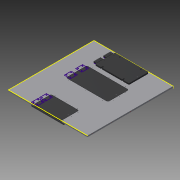
# Autodesk Inventor part: Front_part
Saved by Autodesk Inventor 2015 SP2 (Build 190223200, 223)
## iProperties
Created: 2016-11-11
Part Number: Front_part
Material: Generic
Document SubType Name: Modeling
Designer: Yann Cesbron
Density: 1 g/cm^3
Appearance: Default
Mass: 4194.72 g
Surface Area: 9649.71 cm^2
Volume: 4194.72 cm^3
Material: Perspex Black 9961 -10 mm
Author: Yann Cesbron
Autodesk Inventor part; units mm, degrees
(part 1 of 2)
ref_plane "YZ Plane" through (0, 0, 0) normal (1, 0, 0) x (0, 1, 0)
ref_plane "XZ Plane" through (0, 0, 0) normal (0, 1, 0) x (-1, 0, 0)
ref_plane "XY Plane" through (0, 0, 0) normal (0, 0, 1) x (1, 0, 0)
sketch "Sketch1" plane through (0, 0, 0) normal (0, 0, 1) x (1, 0, 0)
  line L0 (0, 0) -> (565, 0)
  line L1 (565, 0) -> (565, 610)
  line L2 (565, 610) -> (0, 610)
  line L3 (0, 610) -> (0, 0)
  dimension "d0" = 565
  dimension "d1" = 610
  constraints: 8 end point, 2 parallel, 1 horizontal, 1 perpendicular
  measures "d0" distance of L2.end L1.end
  measures "d1" distance of L1.end L0.end
extrude "Extrusion1" add sketch "Sketch1" along normal blind 10
sketch "Cut_out_front" plane through (0, 0, 10) normal (0, 0, 1) x (1, 0, 0)
  line L0 (180, 0) -> (380, 0)
  line L1 (380, 0) -> (380, 115)
  line L2 (370, 125) -> (190, 125)
  line L3 (180, 115) -> (180, 0)
  arc A0 (380, 115) -> (370, 125) centre (370, 115) ccw
  arc A1 (190, 125) -> (180, 115) centre (190, 115) ccw
  line L4 (140, 280) -> (420, 280)
  line L5 (430, 290) -> (430, 420)
  line L6 (420, 430) -> (140, 430)
  line L7 (130, 420) -> (130, 290)
  arc A2 (130, 290) -> (140, 280) centre (140, 290) ccw
  arc A3 (140, 430) -> (130, 420) centre (140, 420) ccw
  arc A4 (430, 420) -> (420, 430) centre (420, 420) ccw
  arc A5 (420, 280) -> (430, 290) centre (420, 290) ccw
  line L8 (0, 610) -> (0, 0) projected
  line L9 (0, 0) -> (565, 0) projected
  line L10 (565, 610) -> (0, 610) projected
  circle A6 centre (117.3, 411.4) radius 1.65
  circle A7 centre (117.3, 379.6) radius 1.65
  circle A8 centre (117.3, 330.4) radius 1.65
  circle A9 centre (117.3, 298.6) radius 1.65
  circle A10 centre (167.3, 13.6) radius 1.65
  circle A11 centre (167.3, 45.4) radius 1.65
  circle A12 centre (167.3, 72.1) radius 1.65
  circle A13 centre (167.3, 103.9) radius 1.65
  line L11 (185, 580) -> (375, 580)
  line L12 (380, 575) -> (380, 485)
  line L13 (375, 480) -> (185, 480)
  line L14 (180, 485) -> (180, 575)
  circle A14 centre (205, 590) radius 2.5
  circle A15 centre (355, 590) radius 2.5
  circle A16 centre (355, 470) radius 2.5
  circle A17 centre (205, 470) radius 2.5
  circle A18 centre (172.5, 565) radius 1.65
  circle A19 centre (172.5, 495) radius 1.65
  circle A20 centre (387.5, 565) radius 1.65
  circle A21 centre (387.5, 495) radius 1.65
  circle A22 centre (122.5, 355) radius 1.65
  circle A23 centre (122.5, 310) radius 1.65
  circle A24 centre (122.5, 400) radius 1.65
  circle A25 centre (160, 272.5) radius 1.65
  circle A26 centre (280, 272.5) radius 1.65
  circle A27 centre (400, 272.5) radius 1.65
  circle A28 centre (437.5, 310) radius 1.65
  circle A29 centre (437.5, 355) radius 1.65
  circle A30 centre (437.5, 400) radius 1.65
  circle A31 centre (400, 437.5) radius 1.65
  circle A32 centre (280, 437.5) radius 1.65
  circle A33 centre (160, 437.5) radius 1.65
  circle A34 centre (172.5, 7.5) radius 1.65
  circle A35 centre (172.5, 62.5) radius 1.65
  circle A36 centre (172.5, 110) radius 1.65
  circle A37 centre (280, 132.5) radius 1.65
  circle A38 centre (387.5, 110) radius 1.65
  circle A39 centre (387.5, 62.5) radius 1.65
  circle A40 centre (387.5, 7.5) radius 1.65
  arc A41 (380, 575) -> (375, 580) centre (375, 575) ccw
  arc A42 (375, 480) -> (380, 485) centre (375, 485) ccw
  arc A43 (180, 485) -> (185, 480) centre (185, 485) ccw
  arc A44 (185, 580) -> (180, 575) centre (185, 575) ccw
  circle A45 centre (200, 132.5) radius 1.65
  circle A46 centre (360, 132.5) radius 1.65
  point P0 (380, 125)
  point P1 (180, 125)
  point P2 (430, 430)
  point P3 (430, 280)
  point P4 (130, 430)
  point P5 (380, 480)
  point P6 (380, 580)
  point P7 (180, 480)
  dimension "d21" = 200
  dimension "d22" = 125
  dimension "d23" = 10
  dimension "d24" = 10
  dimension "d25" = 300
  dimension "d26" = 150
  dimension "d27" = 10
  dimension "d31" = 180
  dimension "d32" = 130
  dimension "d34" = 280
  dimension "d36" = 3.3
  dimension "d37" = 3.3
  dimension "d38" = 3.3
  dimension "d39" = 3.3
  dimension "d40" = 12.7
  dimension "d41" = 12.7
  dimension "d42" = 12.7
  dimension "d43" = 12.7
  dimension "d44" = 31.8
  dimension "d45" = 31.8
  dimension "d87" = 18.6
  dimension "d88" = 18.6
  dimension "d126" = 3.3
  dimension "d127" = 3.3
  dimension "d128" = 3.3
  dimension "d129" = 3.3
  dimension "d130" = 12.7
  dimension "d131" = 12.7
  dimension "d132" = 12.7
  dimension "d133" = 12.7
  dimension "d134" = 21.1
  dimension "d135" = 31.8
  dimension "d136" = 13.6
  dimension "d137" = 31.8
  dimension "d142" = 200
  dimension "d143" = 100
  dimension "d144" = 30
  dimension "d145" = 180
  dimension "d148" = 5
  dimension "d149" = 5
  dimension "d150" = 5
  dimension "d151" = 5
  dimension "d152" = 10
  dimension "d153" = 10
  dimension "d154" = 10
  dimension "d155" = 10
  dimension "d156" = 25
  dimension "d157" = 25
  dimension "d158" = 25
  dimension "d159" = 25
  dimension "d160" = 3.3
  dimension "d161" = 3.3
  dimension "d162" = 3.3
  dimension "d163" = 3.3
  dimension "d164" = 7.5
  dimension "d165" = 7.5
  dimension "d166" = 7.5
  dimension "d167" = 7.5
  dimension "d168" = 15
  dimension "d169" = 15
  dimension "d170" = 15
  dimension "d171" = 15
  dimension "d188" = 3.3
  dimension "d189" = 3.3
  constraints: 47 centre point, 24 end point, 20 point on circle, 20 tangent, 16 point on line, 7 parallel, 6 equal radius, 3 horizontal, 3 perpendicular, 1 collinear
  measures "d21" distance of point (180, 125) point (380, 125)
  measures "d22" distance of point (380, 125) L1.start
  measures "d23" radius of A0
  measures "d24" radius of A1
  measures "d25" distance of point (130, 430) point (430, 430)
  measures "d26" distance of point (430, 430) point (430, 280)
  measures "d27" radius of A2
  measures "d31" distance between parallel lines of L8 L3
  measures "d32" distance between parallel lines of L8 L7
  measures "d34" distance between parallel lines of L9 L4
  measures "d36" diameter of A6
  measures "d37" diameter of A7
  measures "d38" diameter of A8
  measures "d39" diameter of A9
  measures "d40" distance from line of L7 A6.centre
  measures "d41" distance from line of L7 A7.centre
  measures "d42" distance from line of L7 A8.centre
  measures "d43" distance from line of L7 A9.centre
  measures "d44" distance of A7.centre A6.centre
  measures "d45" distance of A9.centre A8.centre
  measures "d87" distance from line of L6 A6.centre
  measures "d88" distance from line of L4 A9.centre
  measures "d126" diameter of A10
  measures "d127" diameter of A11
  measures "d128" diameter of A12
  measures "d129" diameter of A13
  measures "d130" distance from line of L3 A13.centre
  measures "d131" distance from line of L3 A12.centre
  measures "d132" distance from line of L3 A11.centre
  measures "d133" distance from line of L3 A10.centre
  measures "d134" distance from line of L2 A13.centre
  measures "d135" distance of A12.centre A13.centre
  measures "d136" distance from line of L9 A10.centre
  measures "d137" distance of A11.centre A10.centre
  measures "d142" distance of point (380, 480) point (180, 480)
  measures "d143" distance of point (380, 580) point (380, 480)
  measures "d144" distance between parallel lines of L10 L11
  measures "d145" distance between parallel lines of L8 L14
  measures "d148" diameter of A14
  measures "d149" diameter of A15
  measures "d150" diameter of A16
  measures "d151" diameter of A17
  measures "d152" distance from line of L11 A14.centre
  measures "d153" distance from line of L11 A15.centre
  measures "d154" distance from line of L13 A17.centre
  measures "d155" distance from line of L13 A16.centre
  measures "d156" distance from line of A14.centre L14
  measures "d157" distance from line of L12 A15.centre
  measures "d158" distance from line of L12 A16.centre
  measures "d159" distance from line of L14 A17.centre
  measures "d160" diameter of A18
  measures "d161" diameter of A19
  measures "d162" diameter of A20
  measures "d163" diameter of A21
  measures "d164" distance from line of L14 A18.centre
  measures "d165" distance from line of L14 A19.centre
  measures "d166" distance from line of L12 A21.centre
  measures "d167" distance from line of L12 A20.centre
  measures "d168" distance from line of L11 A20.centre
  measures "d169" distance from line of L13 A21.centre
  measures "d170" distance from line of L13 A19.centre
  measures "d171" distance from line of L11 A18.centre
  measures "d188" diameter of A22
  measures "d189" diameter of A23
sketch "Windows_front" plane through (0, 0, 0) normal (0, 0, -1) x (-1, 0, 0)
  line L0 (-395, 585) -> (-165, 585)
  line L1 (-165, 585) -> (-165, 475)
  line L2 (-165, 475) -> (-395, 475)
  line L3 (-395, 585) -> (-165, 475) construction
  line L4 (-165, 585) -> (-395, 475) construction
  line L5 (0, 610) -> (0, 0) projected
  line L6 (-565, 610) -> (0, 610) projected
  line L7 (-395, 535) -> (-385, 535)
  line L8 (-385, 535) -> (-385, 525)
  line L9 (-385, 525) -> (-395, 525)
  line L10 (-395, 475) -> (-395, 525)
  line L11 (-395, 535) -> (-395, 585)
  point P0 (-280, 530)
  dimension "d184" = 230
  dimension "d185" = 110
  dimension "d186" = 280
  dimension "d187" = 80
  dimension "d821" = 10
  dimension "d822" = 50
  dimension "d824" = 10
  dimension "d825" = 10
  constraints: 20 end point, 4 parallel, 2 horizontal, 2 midpoint, 2 perpendicular
  measures "d184" distance of L1.end L2.end
  measures "d185" distance of L0.end L1.end
  measures "d186" distance from line of L5 point (-280, 530)
  measures "d187" distance from line of L6 point (-280, 530)
  measures "d821" distance of L7.end L8.end
  measures "d822" distance between parallel lines of L0 L7
  measures "d824" distance between parallel lines of L11 L8
  measures "d825" distance between parallel lines of L10 L8
sketch "Hinges_middle_bottom_front" plane through (0, 0, 10) normal (0, 0, 1) x (1, 0, 0)
  line L0 (108, 420) -> (152, 420)
  line L1 (152, 420) -> (152, 371)
  line L2 (152, 371) -> (108, 371)
  line L3 (108, 371) -> (108, 420)
  line L4 (108, 290) -> (152, 290)
  line L5 (152, 290) -> (152, 339)
  line L6 (152, 339) -> (108, 339)
  line L7 (108, 339) -> (108, 290)
  line L8 (0, 610) -> (0, 0) projected
  line L9 (0, 0) -> (565, 0) projected
  circle A0 centre (117.3, 411.4) radius 2.25
  circle A1 centre (117.3, 379.6) radius 2.25
  circle A2 centre (117.3, 330.4) radius 2.25
  circle A3 centre (117.3, 298.6) radius 2.25
  circle A4 centre (142.7, 411.4) radius 2.25
  circle A5 centre (142.7, 379.6) radius 2.25
  circle A6 centre (142.7, 330.4) radius 2.25
  circle A7 centre (142.7, 298.6) radius 2.25
  line L10 (158, 112.5) -> (202, 112.5)
  line L11 (202, 112.5) -> (202, 63.5)
  line L12 (202, 63.5) -> (158, 63.5)
  line L13 (158, 63.5) -> (158, 112.5)
  line L14 (158, 54) -> (202, 54)
  line L15 (202, 54) -> (202, 5)
  line L16 (202, 5) -> (158, 5)
  line L17 (158, 5) -> (158, 54)
  circle A8 centre (167.3, 103.9) radius 2.25
  circle A9 centre (167.3, 72.1) radius 2.25
  circle A10 centre (192.7, 103.9) radius 2.25
  circle A11 centre (192.7, 72.1) radius 2.25
  circle A12 centre (167.3, 45.4) radius 2.25
  circle A13 centre (192.7, 45.4) radius 2.25
  circle A14 centre (167.3, 13.6) radius 2.25
  circle A15 centre (192.7, 13.6) radius 2.25
  dimension "d56" = 44
  dimension "d57" = 49
  dimension "d58" = 44
  dimension "d59" = 49
  dimension "d60" = 108
  dimension "d61" = 290
  dimension "d62" = 371
  dimension "d63" = 4.5
  dimension "d64" = 4.5
  dimension "d65" = 4.5
  dimension "d66" = 4.5
  dimension "d67" = 4.5
  dimension "d68" = 4.5
  dimension "d69" = 4.5
  dimension "d70" = 4.5
  dimension "d71" = 9.3
  dimension "d72" = 9.3
  dimension "d73" = 9.3
  dimension "d74" = 9.3
  dimension "d75" = 9.3
  dimension "d76" = 8.6
  dimension "d77" = 8.6
  dimension "d78" = 8.6
  dimension "d79" = 8.6
  dimension "d80" = 8.6
  dimension "d81" = 8.6
  dimension "d82" = 8.6
  dimension "d83" = 8.6
  dimension "d84" = 9.3
  dimension "d85" = 9.3
  dimension "d86" = 9.3
  dimension "d89" = 44
  dimension "d90" = 49
  dimension "d91" = 44
  dimension "d92" = 49
  dimension "d93" = 5
  dimension "d96" = 112.5
  dimension "d100" = 158
  dimension "d101" = 158
  dimension "d102" = 4.5
  dimension "d103" = 4.5
  dimension "d104" = 4.5
  dimension "d105" = 4.5
  dimension "d106" = 4.5
  dimension "d107" = 4.5
  dimension "d108" = 4.5
  dimension "d109" = 4.5
  dimension "d110" = 8.6
  dimension "d111" = 8.6
  dimension "d112" = 8.6
  dimension "d113" = 8.6
  dimension "d114" = 8.6
  dimension "d115" = 8.6
  dimension "d116" = 8.6
  dimension "d117" = 8.6
  dimension "d118" = 9.3
  dimension "d119" = 9.3
  dimension "d120" = 9.3
  dimension "d121" = 9.3
  dimension "d122" = 9.3
  dimension "d123" = 9.3
  dimension "d124" = 9.3
  dimension "d125" = 9.3
  constraints: 32 end point, 16 centre point, 8 parallel, 4 horizontal, 4 perpendicular, 1 point on line
  measures "d56" distance of L1.end L2.end
  measures "d57" distance of L0.end L1.end
  measures "d58" distance of L6.end L5.end
  measures "d59" distance of L5.end L4.end
  measures "d60" distance between parallel lines of L8 L3
  measures "d61" distance between parallel lines of L9 L4
  measures "d62" distance between parallel lines of L9 L2
  measures "d63" diameter of A0
  measures "d64" diameter of A1
  measures "d65" diameter of A2
  measures "d66" diameter of A3
  measures "d67" diameter of A4
  measures "d68" diameter of A5
  measures "d69" diameter of A6
  measures "d70" diameter of A7
  measures "d71" distance from line of L1 A5.centre
  measures "d72" distance from line of L1 A4.centre
  measures "d73" distance from line of L5 A6.centre
  measures "d74" distance from line of L3 A0.centre
  measures "d75" distance from line of L3 A1.centre
  measures "d76" distance from line of L0 A0.centre
  measures "d77" distance from line of L2 A1.centre
  measures "d78" distance from line of L2 A5.centre
  measures "d79" distance from line of L0 A4.centre
  measures "d80" distance from line of L6 A2.centre
  measures "d81" distance from line of L6 A6.centre
  measures "d82" distance from line of L4 A3.centre
  measures "d83" distance from line of L4 A7.centre
  measures "d84" distance from line of L7 A2.centre
  measures "d85" distance from line of L7 A3.centre
  measures "d86" distance from line of L5 A7.centre
  measures "d89" distance of L11.end L12.end
  measures "d90" distance of L10.end L11.end
  measures "d91" distance of L15.end L16.end
  measures "d92" distance of L14.end L15.end
  measures "d93" distance between parallel lines of L9 L16
  measures "d96" distance between parallel lines of L9 L10
  measures "d100" distance between parallel lines of L8 L13
  measures "d101" distance between parallel lines of L8 L17
  measures "d102" diameter of A8
  measures "d103" diameter of A9
  measures "d104" diameter of A10
  measures "d105" diameter of A11
  measures "d106" diameter of A12
  measures "d107" diameter of A13
  measures "d108" diameter of A14
  measures "d109" diameter of A15
  measures "d110" distance from line of L10 A8.centre
  measures "d111" distance from line of L10 A10.centre
  measures "d112" distance from line of L12 A9.centre
  measures "d113" distance from line of L12 A11.centre
  measures "d114" distance from line of A12.centre L14
  measures "d115" distance from line of L14 A13.centre
  measures "d116" distance from line of L16 A14.centre
  measures "d117" distance from line of L16 A15.centre
  measures "d118" distance from line of L13 A9.centre
  measures "d119" distance from line of L13 A8.centre
  measures "d120" distance from line of L11 A10.centre
  measures "d121" distance from line of L11 A11.centre
  measures "d122" distance from line of L15 A13.centre
  measures "d123" distance from line of L15 A15.centre
  measures "d124" distance from line of L17 A14.centre
  measures "d125" distance from line of L17 A12.centre
sketch "Top_door_hinge_levellers_front" plane through (0, 0, 10) normal (0, 0, 1) x (1, 0, 0)
  line L0 (158, 540.5) -> (138, 540.5)
  line L1 (138, 540.5) -> (138, 589.5)
  line L2 (138, 589.5) -> (158, 589.5)
  line L3 (158, 589.5) -> (158, 540.5)
  line L4 (138, 519.5) -> (158, 519.5)
  line L5 (158, 519.5) -> (158, 470.5)
  line L6 (158, 470.5) -> (138, 470.5)
  line L7 (138, 470.5) -> (138, 519.5)
  line L8 (565, 610) -> (0, 610) projected
  line L9 (0, 610) -> (0, 0) projected
  circle A0 centre (147.3, 580.9) radius 1.65
  circle A1 centre (147.3, 549.1) radius 1.65
  circle A2 centre (147.3, 479.1) radius 1.65
  circle A3 centre (147.3, 510.9) radius 1.65
  dimension "d304" = 20
  dimension "d305" = 49
  dimension "d306" = 20
  dimension "d307" = 49
  dimension "d308" = 20.5
  dimension "d309" = 139.5
  dimension "d310" = 138
  dimension "d311" = 138
  dimension "d312" = 3.3
  dimension "d313" = 3.3
  dimension "d314" = 3.3
  dimension "d315" = 3.3
  dimension "d316" = 8.6
  dimension "d317" = 8.6
  dimension "d318" = 9.3
  dimension "d319" = 9.3
  dimension "d320" = 9.3
  dimension "d321" = 9.3
  dimension "d322" = 8.6
  dimension "d323" = 8.6
  constraints: 16 end point, 4 centre point, 4 parallel, 2 horizontal, 2 perpendicular
  measures "d304" distance of L1.end L2.end
  measures "d305" distance of L0.end L1.end
  measures "d306" distance of L5.end L6.end
  measures "d307" distance of L4.end L5.end
  measures "d308" distance between parallel lines of L8 L2
  measures "d309" distance between parallel lines of L6 L8
  measures "d310" distance between parallel lines of L9 L1
  measures "d311" distance between parallel lines of L9 L7
  measures "d312" diameter of A0
  measures "d313" diameter of A1
  measures "d314" diameter of A2
  measures "d315" diameter of A3
  measures "d316" distance from line of L2 A0.centre
  measures "d317" distance from line of L0 A1.centre
  measures "d318" distance from line of L1 A1.centre
  measures "d319" distance from line of A0.centre L1
  measures "d320" distance from line of L7 A2.centre
  measures "d321" distance from line of L7 A3.centre
  measures "d322" distance from line of L4 A3.centre
  measures "d323" distance from line of L6 A2.centre
sketch "Top_door_front" plane through (0, 0, 10) normal (0, 0, 1) x (1, 0, 0)
  line L0 (165, 600) -> (395, 600)
  line L1 (400, 595) -> (400, 465)
  line L2 (160, 465) -> (160, 595)
  line L3 (160, 600) -> (400, 460) construction
  line L4 (400, 600) -> (160, 460) construction
  line L5 (565, 610) -> (0, 610) projected
  line L6 (0, 610) -> (0, 0) projected
  arc A0 (208.5, 470) -> (201.5, 470) centre (205, 470) ccw
  arc A1 (358.5, 470) -> (351.5, 470) centre (355, 470) ccw
  circle A2 centre (355, 590) radius 4
  circle A3 centre (205, 590) radius 4
  line L7 (201.5, 470) -> (201.5, 460)
  line L8 (208.5, 470) -> (208.5, 460)
  line L9 (351.5, 470) -> (351.5, 460)
  line L10 (358.5, 470) -> (358.5, 460)
  line L11 (395, 460) -> (358.5, 460)
  line L12 (351.5, 460) -> (208.5, 460)
  line L13 (201.5, 460) -> (165, 460)
  circle A4 centre (172.7, 580.9) radius 1.65
  circle A5 centre (172.7, 549.1) radius 1.65
  circle A6 centre (172.7, 510.9) radius 1.65
  circle A7 centre (172.7, 479.1) radius 1.65
  arc A8 (400, 595) -> (395, 600) centre (395, 595) ccw
  arc A9 (165, 600) -> (160, 595) centre (165, 595) ccw
  arc A10 (160, 465) -> (165, 460) centre (165, 465) ccw
  arc A11 (395, 460) -> (400, 465) centre (395, 465) ccw
  point P0 (280, 530)
  dimension "d138" = 240
  dimension "d139" = 140
  dimension "d146" = 280
  dimension "d147" = 80
  dimension "d172" = 7
  dimension "d173" = 7
  dimension "d174" = 8
  dimension "d175" = 8
  dimension "d176" = 10
  dimension "d177" = 10
  dimension "d180" = 45
  dimension "d181" = 45
  dimension "d182" = 45
  dimension "d183" = 45
  dimension "d299" = 10
  dimension "d300" = 10
  dimension "d301" = 150
  dimension "d302" = 10
  dimension "d388" = 3.3
  dimension "d389" = 3.3
  dimension "d390" = 3.3
  dimension "d391" = 3.3
  dimension "d392" = 19.1
  dimension "d393" = 31.8
  dimension "d394" = 31.8
  dimension "d395" = 19.1
  dimension "d396" = 12.7
  dimension "d397" = 12.7
  dimension "d398" = 12.7
  dimension "d399" = 12.7
  dimension "d400" = 5
  dimension "d401" = 5
  dimension "d402" = 5
  constraints: 24 end point, 13 perpendicular, 12 centre point, 12 point on circle, 12 tangent, 8 point on line, 4 parallel, 2 midpoint, 1 equal radius, 1 horizontal
  measures "d138" distance of L3.end L4.end
  measures "d139" distance of L4.start L3.end
  measures "d146" distance from line of L6 point (280, 530)
  measures "d147" distance from line of L5 point (280, 530)
  measures "d172" diameter of A0
  measures "d173" diameter of A1
  measures "d174" diameter of A2
  measures "d175" diameter of A3
  measures "d176" distance from line of L0 A2.centre
  measures "d177" distance from line of L0 A3.centre
  measures "d180" distance from line of L2 A3.centre
  measures "d181" distance from line of L1 A2.centre
  measures "d182" distance from line of L1 A1.centre
  measures "d183" distance from line of L2 A0.centre
  measures "d299" distance from line of L12 A1.centre
  measures "d300" distance from line of L12 A0.centre
  measures "d301" distance between parallel lines of L5 L12
  measures "d302" distance between parallel lines of L5 L0
  measures "d388" diameter of A4
  measures "d389" diameter of A5
  measures "d390" diameter of A6
  measures "d391" diameter of A7
  measures "d392" distance from line of L13 A7.centre
  measures "d393" distance of A6.centre A7.centre
  measures "d394" distance of A4.centre A5.centre
  measures "d395" distance from line of L0 A4.centre
  measures "d396" distance from line of L2 A7.centre
  measures "d397" distance from line of L2 A6.centre
  measures "d398" distance from line of L2 A5.centre
  measures "d399" distance from line of L2 A4.centre
  measures "d400" radius of A8
  measures "d401" radius of A9
  measures "d402" radius of A10
sketch "Hinges_top_front" plane through (0, 0, 10) normal (0, 0, 1) x (1, 0, 0)
  line L0 (182, 519.5) -> (182, 470.5)
  circle A0 centre (172.7, 510.9) radius 2.25
  circle A1 centre (172.7, 479.1) radius 2.25
  circle A2 centre (147.3, 479.1) radius 2.25
  circle A3 centre (147.3, 510.9) radius 2.25
  line L1 (182, 470.5) -> (138, 470.5)
  line L2 (138, 470.5) -> (138, 519.5)
  line L3 (138, 519.5) -> (182, 519.5)
  line L4 (182, 589.5) -> (182, 540.5)
  circle A4 centre (172.7, 580.9) radius 2.25
  circle A5 centre (172.7, 549.1) radius 2.25
  circle A6 centre (147.3, 549.1) radius 2.25
  circle A7 centre (147.3, 580.9) radius 2.25
  line L5 (182, 540.5) -> (138, 540.5)
  line L6 (138, 540.5) -> (138, 589.5)
  line L7 (138, 589.5) -> (182, 589.5)
  line L8 (0, 610) -> (0, 0) projected
  line L9 (565, 610) -> (0, 610) projected
  dimension "d356" = 44
  dimension "d357" = 49
  dimension "d358" = 4.5
  dimension "d359" = 4.5
  dimension "d360" = 4.5
  dimension "d361" = 4.5
  dimension "d362" = 9.3
  dimension "d363" = 9.3
  dimension "d364" = 9.3
  dimension "d365" = 9.3
  dimension "d366" = 8.6
  dimension "d367" = 8.6
  dimension "d368" = 8.6
  dimension "d369" = 8.6
  dimension "d370" = 44
  dimension "d371" = 49
  dimension "d372" = 4.5
  dimension "d373" = 4.5
  dimension "d374" = 4.5
  dimension "d375" = 4.5
  dimension "d376" = 9.3
  dimension "d377" = 9.3
  dimension "d378" = 9.3
  dimension "d379" = 9.3
  dimension "d380" = 8.6
  dimension "d381" = 8.6
  dimension "d382" = 8.6
  dimension "d383" = 8.6
  dimension "d384" = 138
  dimension "d385" = 138
  dimension "d386" = 20.5
  dimension "d387" = 139.5
  constraints: 16 end point, 8 centre point, 4 parallel, 2 horizontal, 2 perpendicular
  measures "d356" distance of L2.end L0.start
  measures "d357" distance of L1.end L2.end
  measures "d358" diameter of A0
  measures "d359" diameter of A1
  measures "d360" diameter of A2
  measures "d361" diameter of A3
  measures "d362" distance from line of L0 A1.centre
  measures "d363" distance from line of L0 A0.centre
  measures "d364" distance from line of L2 A3.centre
  measures "d365" distance from line of A2.centre L2
  measures "d366" distance from line of L1 A2.centre
  measures "d367" distance from line of L1 A1.centre
  measures "d368" distance from line of L3 A0.centre
  measures "d369" distance from line of L3 A3.centre
  measures "d370" distance of L6.end L4.start
  measures "d371" distance of L5.end L6.end
  measures "d372" diameter of A4
  measures "d373" diameter of A5
  measures "d374" diameter of A6
  measures "d375" diameter of A7
  measures "d376" distance from line of L4 A5.centre
  measures "d377" distance from line of L4 A4.centre
  measures "d378" distance from line of L6 A7.centre
  measures "d379" distance from line of A6.centre L6
  measures "d380" distance from line of L5 A6.centre
  measures "d381" distance from line of L5 A5.centre
  measures "d382" distance from line of L7 A4.centre
  measures "d383" distance from line of L7 A7.centre
  measures "d384" distance between parallel lines of L8 L2
  measures "d385" distance between parallel lines of L8 L6
  measures "d386" distance between parallel lines of L9 L7
  measures "d387" distance between parallel lines of L9 L1
sketch "Middle_door_front" plane through (0, 0, 10) normal (0, 0, 1) x (1, 0, 0)
  line L0 (140, 282) -> (420, 282)
  line L1 (428, 290) -> (428, 420)
  line L2 (420, 428) -> (140, 428)
  line L3 (132, 420) -> (132, 290)
  line L4 (132, 282) -> (428, 428) construction
  line L5 (428, 282) -> (132, 428) construction
  line L6 (0, 0) -> (565, 0) projected
  line L7 (0, 610) -> (0, 0) projected
  arc A0 (428, 420) -> (420, 428) centre (420, 420) ccw
  arc A1 (140, 428) -> (132, 420) centre (140, 420) ccw
  arc A2 (132, 290) -> (140, 282) centre (140, 290) ccw
  arc A3 (420, 282) -> (428, 290) centre (420, 290) ccw
  circle A4 centre (142.7, 411.4) radius 1.65
  circle A5 centre (142.7, 379.6) radius 1.65
  circle A6 centre (142.7, 330.4) radius 1.65
  circle A7 centre (142.7, 298.6) radius 1.65
  point P0 (280, 355)
  dimension "d421" = 296
  dimension "d422" = 146
  dimension "d423" = 355
  dimension "d424" = 280
  dimension "d425" = 8
  dimension "d426" = 3.3
  dimension "d427" = 3.3
  dimension "d428" = 3.3
  dimension "d429" = 3.3
  dimension "d430" = 10.7
  dimension "d431" = 10.7
  dimension "d432" = 10.7
  dimension "d433" = 10.7
  dimension "d434" = 31.8
  dimension "d435" = 31.8
  dimension "d436" = 16.6
  dimension "d437" = 16.6
  constraints: 12 end point, 8 centre point, 8 point on circle, 8 point on line, 8 tangent, 3 equal radius, 2 midpoint, 2 parallel, 1 horizontal, 1 perpendicular
  measures "d421" distance of L5.end L4.end
  measures "d422" distance of L4.end L5.start
  measures "d423" distance from line of L6 point (280, 355)
  measures "d424" distance from line of L7 point (280, 355)
  measures "d425" radius of A0
  measures "d426" diameter of A4
  measures "d427" diameter of A5
  measures "d428" diameter of A6
  measures "d429" diameter of A7
  measures "d430" distance from line of L3 A4.centre
  measures "d431" distance from line of L3 A5.centre
  measures "d432" distance from line of L3 A6.centre
  measures "d433" distance from line of L3 A7.centre
  measures "d434" distance of A5.centre A4.centre
  measures "d435" distance of A7.centre A6.centre
  measures "d436" distance from line of L0 A7.centre
  measures "d437" distance from line of L2 A4.centre
sketch "Bottom_door_front" plane through (0, 0, 10) normal (0, 0, 1) x (1, 0, 0)
  line L0 (190, 123) -> (370, 123)
  line L1 (378, 115) -> (378, 2)
  line L2 (378, 2) -> (182, 2)
  line L3 (182, 2) -> (182, 115)
  line L4 (182, 123) -> (378, 2) construction
  line L5 (378, 123) -> (182, 2) construction
  line L6 (0, 610) -> (0, 0) projected
  line L7 (0, 0) -> (565, 0) projected
  arc A0 (378, 115) -> (370, 123) centre (370, 115) ccw
  arc A1 (190, 123) -> (182, 115) centre (190, 115) ccw
  circle A2 centre (192.7, 103.9) radius 1.65
  circle A3 centre (192.7, 72.1) radius 1.65
  circle A4 centre (192.7, 45.4) radius 1.65
  circle A5 centre (192.7, 13.6) radius 1.65
  point P0 (280, 62.5)
  dimension "d404" = 196
  dimension "d405" = 121
  dimension "d406" = 280
  dimension "d407" = 62.5
  dimension "d408" = 8
  dimension "d409" = 3.3
  dimension "d410" = 3.3
  dimension "d411" = 3.3
  dimension "d412" = 3.3
  dimension "d413" = 10.7
  dimension "d414" = 10.7
  dimension "d415" = 10.7
  dimension "d416" = 10.7
  dimension "d417" = 31.8
  dimension "d418" = 31.8
  dimension "d419" = 11.6
  dimension "d420" = 19.1
  constraints: 12 end point, 6 centre point, 4 point on circle, 4 point on line, 4 tangent, 2 midpoint, 2 parallel, 1 equal radius, 1 horizontal, 1 perpendicular
  measures "d404" distance of L1.end L2.end
  measures "d405" distance of L5.start L1.end
  measures "d406" distance from line of L6 point (280, 62.5)
  measures "d407" distance from line of L7 point (280, 62.5)
  measures "d408" radius of A0
  measures "d409" diameter of A2
  measures "d410" diameter of A3
  measures "d411" diameter of A4
  measures "d412" diameter of A5
  measures "d413" distance from line of L3 A2.centre
  measures "d414" distance from line of L3 A3.centre
  measures "d415" distance from line of L3 A4.centre
  measures "d416" distance from line of L3 A5.centre
  measures "d417" distance of A4.centre A5.centre
  measures "d418" distance of A2.centre A3.centre
  measures "d419" distance from line of L2 A5.centre
  measures "d420" distance from line of L0 A2.centre
sketch "Panel_holes_top_front" plane through (0, 610, 0) normal (0, 1, 0) x (1, 0, 0)
  circle A0 centre (30, -5) radius 1.65
  circle A1 centre (535, -5) radius 1.65
  circle A2 centre (195, -5) radius 1.65
  circle A3 centre (370, -5) radius 1.65
  line L0 (565, 0) -> (0, 0) projected
  line L1 (565, -10) -> (0, -10) projected
  line L2 (0, 0) -> (0, -10) projected
  line L3 (565, 0) -> (565, -10) projected
  dimension "d438" = 3.3
  dimension "d439" = 3.3
  dimension "d440" = 3.3
  dimension "d441" = 3.3
  dimension "d442" = 5
  dimension "d443" = 5
  dimension "d444" = 5
  dimension "d445" = 5
  dimension "d446" = 30
  dimension "d447" = 30
  dimension "d448" = 165
  dimension "d449" = 165
  dimension "d450" = 175
  constraints: 4 centre point
  measures "d438" diameter of A0
  measures "d439" diameter of A1
  measures "d440" diameter of A2
  measures "d441" diameter of A3
  measures "d442" distance from line of L0 A0.centre
  measures "d443" distance from line of L1 A2.centre
  measures "d444" distance from line of L1 A3.centre
  measures "d445" distance from line of L1 A1.centre
  measures "d446" distance from line of L2 A0.centre
  measures "d447" distance from line of A1.centre L3
  measures "d448" distance of A0.centre A2.centre
  measures "d449" distance of A3.centre A1.centre
  measures "d450" distance of A3.centre A2.centre
sketch "Panel_holes_right_front" plane through (565, 0, 0) normal (1, 0, 0) x (0, 0, -1)
  circle A0 centre (-5, 575) radius 1.65
  line L0 (0, 0) -> (0, 610) projected
  circle A1 centre (-5, 440) radius 1.65
  circle A2 centre (-5, 305) radius 1.65
  circle A3 centre (-5, 170) radius 1.65
  circle A4 centre (-5, 35) radius 1.65
  line L1 (0, 610) -> (-10, 610) projected
  line L2 (0, 0) -> (-10, 0) projected
  dimension "d451" = 3.3
  dimension "d452" = 5
  dimension "d453" = 3.3
  dimension "d454" = 3.3
  dimension "d455" = 3.3
  dimension "d456" = 3.3
  dimension "d457" = 5
  dimension "d458" = 5
  dimension "d459" = 5
  dimension "d460" = 5
  dimension "d461" = 35
  dimension "d462" = 35
  dimension "d463" = 135
  dimension "d464" = 135
  dimension "d465" = 135
  constraints: 5 centre point
  measures "d451" diameter of A0
  measures "d452" distance from line of L0 A0.centre
  measures "d453" diameter of A1
  measures "d454" diameter of A2
  measures "d455" diameter of A3
  measures "d456" diameter of A4
  measures "d457" distance from line of L0 A4.centre
  measures "d458" distance from line of L0 A3.centre
  measures "d459" distance from line of L0 A2.centre
  measures "d460" distance from line of L0 A1.centre
  measures "d461" distance from line of L1 A0.centre
  measures "d462" distance from line of L2 A4.centre
  measures "d463" distance of A0.centre A1.centre
  measures "d464" distance of A3.centre A4.centre
  measures "d465" distance of A2.centre A3.centre
sketch "Panel_holes_left_front" plane through (0, 0, 0) normal (-1, 0, 0) x (0, 0, 1)
  circle A0 centre (5, 575) radius 1.65
  circle A1 centre (5, 440) radius 1.65
  circle A2 centre (5, 305) radius 1.65
  circle A3 centre (5, 170) radius 1.65
  circle A4 centre (5, 35) radius 1.65
  line L0 (0, 0) -> (0, 610) projected
  line L1 (0, 0) -> (10, 0) projected
  line L2 (0, 610) -> (10, 610) projected
  dimension "d466" = 3.3
  dimension "d467" = 3.3
  dimension "d468" = 3.3
  dimension "d469" = 3.3
  dimension "d470" = 3.3
  dimension "d471" = 5
  dimension "d472" = 35
  dimension "d473" = 5
  dimension "d474" = 135
  dimension "d475" = 5
  dimension "d476" = 135
  dimension "d477" = 5
  dimension "d478" = 5
  dimension "d479" = 35
  dimension "d480" = 135
  constraints: 5 centre point
  measures "d466" diameter of A0
  measures "d467" diameter of A1
  measures "d468" diameter of A2
  measures "d469" diameter of A3
  measures "d470" diameter of A4
  measures "d471" distance from line of L0 A4.centre
  measures "d472" distance from line of L1 A4.centre
  measures "d473" distance from line of L0 A3.centre
  measures "d474" distance of A4.centre A3.centre
  measures "d475" distance from line of L0 A2.centre
  measures "d476" distance of A3.centre A2.centre
  measures "d477" distance from line of L0 A0.centre
  measures "d478" distance from line of L0 A1.centre
  measures "d479" distance from line of L2 A0.centre
  measures "d480" distance of A0.centre A1.centre
extrude "Extrusion2" cut sketch "Cut_out_front" against normal blind 10
extrude "Extrusion3" add sketch "Top_door_front" along normal blind 10 separate body
extrude "Extrusion4" add sketch "Middle_door_front" against normal blind 10 separate body
extrude "Extrusion5" add sketch "Bottom_door_front" against normal blind 10 separate body
extrude "Extrusion6" add sketch "Top_door_hinge_levellers_front" along normal blind 10 separate body
extrude "Extrusion7" add sketch "Windows_front" along normal blind 10 separate body
extrude "Extrusion8" cut sketch "Panel_holes_right_front" against normal blind 15 bodies 1
extrude "Extrusion9" cut sketch "Panel_holes_left_front" against normal blind 15 bodies 1
extrude "Extrusion10" cut sketch "Panel_holes_top_front" against normal blind 15 contours A0 | A1 | A2 | A3 bodies 1
sketch "Bottom_door_hole_front" plane through (0, 0, 0) normal (0, 0, -1) x (-1, 0, 0)
  line L0 (-378, 2) -> (-182, 2) projected
  line L1 (-378, 115) -> (-378, 2) projected
  point P0 (0, 0)
  point P1 (-365, 62.5)
  dimension "d507" = 60.5
  dimension "d508" = 13
  measures "d507" distance from line of L0 point (-365, 62.5)
  measures "d508" distance from line of L1 point (-365, 62.5)
sketch "Middle_door_hole_front" plane through (0, 0, 0) normal (0, 0, -1) x (-1, 0, 0)
  line L0 (-428, 420) -> (-428, 290) projected
  line L1 (-420, 282) -> (-140, 282) projected
  point P0 (0, 0)
  point P1 (-415, 355)
  dimension "d505" = 13
  dimension "d506" = 73
  measures "d505" distance from line of L0 point (-415, 355)
  measures "d506" distance from line of L1 point (-415, 355)
sketch "Top_door_hole_front" plane through (0, 0, 10) normal (0, 0, -1) x (-1, 0, 0)
  line L0 (-400, 465) -> (-400, 595) projected
  line L1 (-358.5, 460) -> (-395, 460) projected
  point P0 (0, 0)
  point P1 (-390, 530)
  dimension "d509" = 10
  dimension "d510" = 70
  measures "d509" distance from line of L0 point (-390, 530)
  measures "d510" distance from line of L1 point (-390, 530)
hole "CSK_Bottom_door_hole_front" at (365, 62.5, 0) direction (0, 0, 1) diameter 7 end through all countersink diameter 12.6 countersink angle 90 bodies 4 clearance for "Countersunk Flat Head Screw DIN EN ISO 2009" size "M6" standard "DIN"
hole "CSK_Middle_door_hole_front" at (415, 355, 0) direction (0, 0, 1) diameter 7 end through all countersink diameter 12.6 countersink angle 90 bodies 3 clearance for "Countersunk Flat Head Screw DIN EN ISO 2009" size "M6" standard "DIN"
hole "CSK_Top_door_hole_front" at (390, 530, 10) direction (0, 0, 1) diameter 7 end through all countersink diameter 12.6 countersink angle 90 bodies 2 clearance for "Countersunk Flat Head Screw DIN EN ISO 2009" size "M6" standard "DIN"
sketch "Middle door_flanges_front" plane through (0, 0, 0) normal (0, 0, -1) x (-1, 0, 0)
  line L0 (-140, 445) -> (-115, 445)
  line L1 (-115, 445) -> (-115, 265)
  line L2 (-115, 265) -> (-140, 265)
  line L3 (-140, 265) -> (-140, 445)
  line L4 (-420, 445) -> (-445, 445)
  line L5 (-445, 445) -> (-445, 265)
  line L6 (-445, 265) -> (-420, 265)
  line L7 (-430, 290) -> (-430, 420) projected
  line L8 (-130, 420) -> (-130, 290) projected
  line L9 (-420, 430) -> (-140, 430) projected
  line L10 (-140, 280) -> (-420, 280) projected
  line L11 (-419, 445) -> (-141, 445)
  line L12 (-141, 445) -> (-141, 420)
  line L13 (-141, 420) -> (-419, 420)
  line L14 (-419, 420) -> (-419, 445)
  line L15 (-419, 290) -> (-141, 290)
  line L16 (-141, 290) -> (-141, 265)
  line L17 (-141, 265) -> (-419, 265)
  line L18 (-419, 265) -> (-419, 290)
  circle A0 centre (-400, 437.5) radius 2.25
  circle A1 centre (-280, 437.5) radius 2.25
  circle A2 centre (-160, 437.5) radius 2.25
  circle A3 centre (-437.5, 400) radius 2.25
  circle A4 centre (-437.5, 355) radius 2.25
  circle A5 centre (-437.5, 310) radius 2.25
  circle A6 centre (-400, 272.5) radius 2.25
  circle A7 centre (-280, 272.5) radius 2.25
  circle A8 centre (-160, 272.5) radius 2.25
  circle A9 centre (-122.5, 310) radius 2.25
  circle A10 centre (-122.5, 355) radius 2.25
  circle A11 centre (-122.5, 400) radius 2.25
  line L19 (-428, 365) -> (-420, 365)
  line L20 (-420, 345) -> (-428, 345)
  line L21 (-428, 345) -> (-428, 365)
  line L22 (-420, 265) -> (-420, 345)
  line L23 (-420, 365) -> (-420, 445)
  circle A12 centre (-427.5, 372.5) radius 1.65
  circle A13 centre (-427.5, 337.5) radius 1.65
  point P0 (0, 0)
  dimension "d533" = 10
  dimension "d537" = 25
  dimension "d538" = 180
  dimension "d539" = 15
  dimension "d540" = 15
  dimension "d543" = 25
  dimension "d544" = 278
  dimension "d545" = 1
  dimension "d546" = 15
  dimension "d547" = 25
  dimension "d548" = 278
  dimension "d549" = 4.5
  dimension "d550" = 4.5
  dimension "d551" = 4.5
  dimension "d552" = 4.5
  dimension "d553" = 4.5
  dimension "d554" = 4.5
  dimension "d555" = 4.5
  dimension "d556" = 4.5
  dimension "d557" = 4.5
  dimension "d558" = 4.5
  dimension "d559" = 4.5
  dimension "d560" = 4.5
  dimension "d561" = 7.5
  dimension "d562" = 7.5
  dimension "d563" = 7.5
  dimension "d564" = 7.5
  dimension "d565" = 7.5
  dimension "d566" = 19
  dimension "d567" = 45
  dimension "d568" = 45
  dimension "d569" = 19
  dimension "d570" = 7.5
  dimension "d571" = 7.5
  dimension "d572" = 45
  dimension "d573" = 120
  dimension "d574" = 19
  dimension "d575" = 7.5
  dimension "d576" = 45
  dimension "d577" = 7.5
  dimension "d578" = 7.5
  dimension "d579" = 7.5
  dimension "d580" = 7.5
  dimension "d581" = 19
  dimension "d582" = 45
  dimension "d583" = 45
  dimension "d584" = 120
  dimension "d589" = 1
  dimension "d590" = 8
  dimension "d591" = 20
  dimension "d592" = 25
  dimension "d593" = 25
  dimension "d594" = 80
  dimension "d595" = 10
  dimension "d596" = 3.3
  dimension "d597" = 3.3
  dimension "d598" = 7.5
  dimension "d599" = 7.5
  dimension "d600" = 7.5
  dimension "d601" = 7.5
  constraints: 40 end point, 14 centre point, 10 parallel, 5 horizontal, 4 perpendicular, 2 point on line
  measures "d533" distance between parallel lines of L8 L3
  measures "d537" distance between parallel lines of L1 L3
  measures "d538" distance between parallel lines of L0 L2
  measures "d539" distance between parallel lines of L10 L2
  measures "d540" distance between parallel lines of L9 L11
  measures "d543" distance between parallel lines of L11 L13
  measures "d544" distance between parallel lines of L14 L12
  measures "d545" distance between parallel lines of L3 L16
  measures "d546" distance between parallel lines of L10 L17
  measures "d547" distance between parallel lines of L17 L15
  measures "d548" distance between parallel lines of L18 L16
  measures "d549" diameter of A0
  measures "d550" diameter of A1
  measures "d551" diameter of A2
  measures "d552" diameter of A3
  measures "d553" diameter of A4
  measures "d554" diameter of A5
  measures "d555" diameter of A6
  measures "d556" diameter of A7
  measures "d557" diameter of A8
  measures "d558" diameter of A9
  measures "d559" diameter of A10
  measures "d560" diameter of A11
  measures "d561" distance from line of L11 A2.centre
  measures "d562" distance from line of L1 A11.centre
  measures "d563" distance from line of L1 A10.centre
  measures "d564" distance from line of L1 A9.centre
  measures "d565" distance from line of L11 A1.centre
  measures "d566" distance from line of L12 A2.centre
  measures "d567" distance from line of L0 A11.centre
  measures "d568" distance from line of L2 A9.centre
  measures "d569" distance from line of L16 A8.centre
  measures "d570" distance from line of L17 A8.centre
  measures "d571" distance from line of L17 A7.centre
  measures "d572" distance of A10.centre A9.centre
  measures "d573" distance of A7.centre A8.centre
  measures "d574" distance from line of L18 A6.centre
  measures "d575" distance from line of L17 A6.centre
  measures "d576" distance from line of A5.centre L6
  measures "d577" distance from line of L5 A4.centre
  measures "d578" distance from line of L5 A5.centre
  measures "d579" distance from line of L5 A3.centre
  measures "d580" distance from line of L11 A0.centre
  measures "d581" distance from line of L14 A0.centre
  measures "d582" distance from line of L4 A3.centre
  measures "d583" distance of A3.centre A4.centre
  measures "d584" distance of A0.centre A1.centre
  measures "d589" distance between parallel lines of L23 L14
  measures "d590" distance between parallel lines of L23 L21
  measures "d591" distance between parallel lines of L19 L20
  measures "d592" distance between parallel lines of L22 L5
  measures "d593" distance between parallel lines of L5 L23
  measures "d594" distance between parallel lines of L19 L4
  measures "d595" distance between parallel lines of L7 L22
  measures "d596" diameter of A12
  measures "d597" diameter of A13
  measures "d598" distance from line of L23 A12.centre
  measures "d599" distance from line of L19 A12.centre
  measures "d600" distance from line of L20 A13.centre
  measures "d601" distance from line of L22 A13.centre
extrude "Middle door_flanges_front_1" add sketch "Middle door_flanges_front" along normal blind 10 separate body contours L0 L1 L2 L3
extrude "Middle door_flanges_front_2" add sketch "Middle door_flanges_front" along normal blind 10 separate body contours L16 L17 L18 L10 | L10 L18 L15 L16
extrude "Middle door_flanges_front_3" add sketch "Middle door_flanges_front" along normal blind 10 separate body contours L12 L13 L14 L9 | L9 L14 L11 L12
extrude "Middle door_flanges_front_4" add sketch "Middle door_flanges_front" along normal blind 10 separate body contours L23 L19 L21 L20 L22 L6 L5 L4
sketch "Bottom_door_flanges_front" plane through (0, 0, 0) normal (0, 0, -1) x (-1, 0, 0)
  line L0 (-370, 125) -> (-190, 125) projected
  line L1 (-165, 140) -> (-190, 140)
  line L2 (-190, 140) -> (-190, 16)
  line L3 (-190, 16) -> (-165, 16)
  line L4 (-165, 16) -> (-165, 140)
  line L5 (-180, 115) -> (-180, 0) projected
  circle A0 centre (-387.5, 110) radius 2.25
  circle A1 centre (-387.5, 62.5) radius 2.25
  circle A2 centre (-387.5, 7.5) radius 2.25
  circle A3 centre (-172.5, 110) radius 2.25
  circle A4 centre (-172.5, 62.5) radius 2.25
  circle A5 centre (-172.5, 7.5) radius 2.25
  line L6 (-191, 115) -> (-369, 115)
  line L7 (-369, 115) -> (-369, 140)
  line L8 (-369, 140) -> (-191, 140)
  line L9 (-191, 140) -> (-191, 115)
  line L10 (-395, 0) -> (-165, 0)
  line L11 (-165, 0) -> (-165, 15)
  line L12 (-165, 15) -> (-395, 15)
  line L13 (-395, 15) -> (-395, 0)
  line L14 (-380, 0) -> (-565, 0) projected
  line L15 (-395, 140) -> (-370, 140)
  line L16 (-370, 16) -> (-395, 16)
  line L17 (-395, 16) -> (-395, 140)
  line L18 (-380, 0) -> (-380, 115) projected
  circle A6 centre (-360, 132.5) radius 2.25
  circle A7 centre (-280, 132.5) radius 2.25
  circle A8 centre (-200, 132.5) radius 2.25
  line L19 (-378, 72.5) -> (-370, 72.5)
  line L20 (-370, 52.5) -> (-378, 52.5)
  line L21 (-378, 52.5) -> (-378, 72.5)
  line L22 (-370, 140) -> (-370, 72.5)
  line L23 (-370, 52.5) -> (-370, 16)
  circle A9 centre (-377.5, 80) radius 1.65
  circle A10 centre (-377.5, 45) radius 1.65
  dimension "d614" = 25
  dimension "d615" = 15
  dimension "d617" = 4.5
  dimension "d618" = 4.5
  dimension "d620" = 4.5
  dimension "d621" = 4.5
  dimension "d622" = 4.5
  dimension "d627" = 7.5
  dimension "d628" = 7.5
  dimension "d634" = 47.5
  dimension "d639" = 178
  dimension "d641" = 15
  dimension "d642" = 15
  dimension "d643" = 25
  dimension "d652" = 124
  dimension "d653" = 1
  dimension "d654" = 1
  dimension "d655" = 230
  dimension "d656" = 15
  dimension "d657" = 46.5
  dimension "d658" = 7.5
  dimension "d659" = 7.5
  dimension "d660" = 30
  dimension "d661" = 25
  dimension "d662" = 124
  dimension "d665" = 30
  dimension "d666" = 7.5
  dimension "d667" = 7.5
  dimension "d668" = 7.5
  dimension "d670" = 1
  dimension "d671" = 7.5
  dimension "d672" = 4.5
  dimension "d673" = 4.5
  dimension "d674" = 4.5
  dimension "d675" = 7.5
  dimension "d676" = 7.5
  dimension "d677" = 7.5
  dimension "d678" = 9
  dimension "d679" = 80
  dimension "d680" = 9
  dimension "d686" = 25
  dimension "d687" = 1
  dimension "d688" = 20
  dimension "d689" = 67.5
  dimension "d690" = 8
  dimension "d691" = 3.3
  dimension "d692" = 3.3
  dimension "d693" = 7.5
  dimension "d694" = 7.5
  dimension "d695" = 7.5
  dimension "d696" = 7.5
  constraints: 40 end point, 11 centre point, 10 parallel, 5 horizontal, 5 perpendicular, 1 collinear, 1 equal radius
  measures "d614" distance of L3.end L2.end
  measures "d615" distance between parallel lines of L5 L4
  measures "d617" diameter of A0
  measures "d618" diameter of A1
  measures "d620" diameter of A3
  measures "d621" diameter of A4
  measures "d622" diameter of A5
  measures "d627" distance from line of L4 A4.centre
  measures "d628" distance from line of L4 A3.centre
  measures "d634" distance of A0.centre A1.centre
  measures "d639" distance between parallel lines of L7 L9
  measures "d641" distance between parallel lines of L12 L10
  measures "d642" distance between parallel lines of L8 L0
  measures "d643" distance between parallel lines of L8 L6
  measures "d652" distance between parallel lines of L3 L1
  measures "d653" distance between parallel lines of L9 L2
  measures "d654" distance between parallel lines of L12 L3
  measures "d655" distance between parallel lines of L13 L11
  measures "d656" distance between parallel lines of L5 L11
  measures "d657" distance from line of L3 A4.centre
  measures "d658" distance from line of L11 A5.centre
  measures "d659" distance from line of L10 A5.centre
  measures "d660" distance from line of L1 A3.centre
  measures "d661" distance of L16.start L16.end
  measures "d662" distance of L15.end L16.start
  measures "d665" distance from line of L15 A0.centre
  measures "d666" distance from line of L17 A0.centre
  measures "d667" distance from line of L17 A1.centre
  measures "d668" distance from line of L10 A2.centre
  measures "d670" distance between parallel lines of L16 L12
  measures "d671" distance from line of A2.centre L13
  measures "d672" diameter of A6
  measures "d673" diameter of A7
  measures "d674" diameter of A8
  measures "d675" distance from line of L8 A6.centre
  measures "d676" distance from line of L8 A7.centre
  measures "d677" distance from line of L8 A8.centre
  measures "d678" distance from line of L9 A8.centre
  measures "d679" distance of A8.centre A7.centre
  measures "d680" distance from line of L7 A6.centre
  measures "d686" distance between parallel lines of L22 L17
  measures "d687" distance between parallel lines of L7 L22
  measures "d688" distance between parallel lines of L20 L19
  measures "d689" distance between parallel lines of L15 L19
  measures "d690" distance between parallel lines of L23 L21
  measures "d691" diameter of A9
  measures "d692" diameter of A10
  measures "d693" distance from line of L22 A9.centre
  measures "d694" distance from line of L19 A9.centre
  measures "d695" distance from line of L20 A10.centre
  measures "d696" distance from line of L23 A10.centre
extrude "Bottom_door_flanges_front_1" add sketch "Bottom_door_flanges_front" along normal blind 10 separate body contours L2 L1 L4 L3
extrude "Bottom_door_flanges_front_2" add sketch "Bottom_door_flanges_front" along normal blind 10 separate body contours L7 L8 L9 L0 | L0 L9 L6 L7
extrude "Bottom_door_flanges_front_3" add sketch "Bottom_door_flanges_front" along normal blind 10 separate body contours L18 L10 L13 L12 | L12 L5 L10 L18 | L12 L11 L10 L5
extrude "Bottom_door_flanges_front_4" add sketch "Bottom_door_flanges_front" along normal blind 10 separate body contours L22 L19 L21 L20 L23 L16 L17 L15